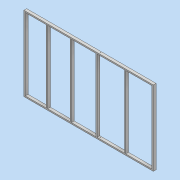
# Autodesk Inventor part: Khung cửa
Saved by Autodesk Inventor 2018 (Build 220112000, 112)
## iProperties
Created: 2020-08-10
Part Number: Khung cửa
Material: Generic
Document SubType Name: Modeling
Designer: ASUS
Density: 1 g/cm^3
Appearance: Default
Author: ASUS
Autodesk Inventor part; units mm, degrees
ref_plane "YZ Plane" through (0, 0, 0) normal (1, 0, 0) x (0, 1, 0)
ref_plane "XZ Plane" through (0, 0, 0) normal (0, 1, 0) x (-1, 0, 0)
ref_plane "XY Plane" through (0, 0, 0) normal (0, 0, 1) x (1, 0, 0)
sketch "Sketch1" plane through (0, 0, 0) normal (0, 1, 0) x (-1, 0, 0)
  line L0 (0, 0) -> (2835, 0)
  line L1 (2835, 0) -> (2835, -1640)
  line L2 (2835, -1640) -> (0, -1640)
  line L3 (0, -1640) -> (0, 0)
  line L4 (30, -30) -> (30, -1610)
  line L5 (2805, -1610) -> (2805, -30)
  line L6 (1232.5, -30) -> (1232.5, -1610)
  line L7 (1262.5, -1610) -> (1262.5, -30)
  line L8 (605, -30) -> (605, -1610)
  line L9 (635, -1610) -> (635, -30)
  line L10 (2315, -30) -> (2315, -1610)
  line L11 (2345, -1610) -> (2345, -30)
  line L12 (1825, -30) -> (1825, -1610)
  line L13 (1795, -1610) -> (1795, -30)
  line L14 (605, -30) -> (30, -30)
  line L15 (30, -1610) -> (605, -1610)
  line L16 (635, -1610) -> (1232.5, -1610)
  line L17 (1232.5, -30) -> (635, -30)
  line L18 (1795, -30) -> (1262.5, -30)
  line L19 (1262.5, -1610) -> (1795, -1610)
  line L20 (2805, -30) -> (2345, -30)
  line L21 (2315, -30) -> (1825, -30)
  line L22 (1825, -1610) -> (2315, -1610)
  line L23 (2345, -1610) -> (2805, -1610)
  dimension "d0" = 2835
  dimension "d1" = 1640
  dimension "d3" = 30
  dimension "d5" = 30
  dimension "d6" = 30
  dimension "d7" = 1262.5
  dimension "d8" = 30
  dimension "d9" = 635
  dimension "d10" = 30
  dimension "d11" = 30
  dimension "d12" = 520
  dimension "d13" = 1040
  constraints: 48 end point, 32 parallel, 6 horizontal, 6 perpendicular
  measures "d0" distance of L1.end L2.end
  measures "d1" distance of L0.end L1.end
  measures "d3" distance between parallel lines of L1 L5
  measures "d5" distance between parallel lines of L3 L4
  measures "d6" distance between parallel lines of L6 L7
  measures "d7" distance between parallel lines of L3 L7
  measures "d8" distance between parallel lines of L8 L9
  measures "d9" distance between parallel lines of L3 L9
  measures "d10" distance of L11.start L10.end
  measures "d11" distance between parallel lines of L13 L12
  measures "d12" distance between parallel lines of L1 L10
  measures "d13" distance between parallel lines of L13 L1
extrude "Extrusion1" add sketch "Sketch1" along normal blind 60
sketch "Sketch2" plane through (-2835, 0, 0) normal (0, 0, 1) x (1, 0, 0)
  circle A0 centre (1642.5, 30) radius 5
  line L0 (2835, 0) -> (0, 0) projected
  point P0 (1602.5, 60)
  dimension "d16" = 10
  dimension "d17" = 30
  dimension "d18" = 40
  constraints: 1 centre point
  measures "d16" diameter of A0
  measures "d17" distance from line of L0 A0.centre
  measures "d18" horizontal distance of point (1602.5, 60) A0.centre
extrude "Extrusion2" cut sketch "Sketch2" against normal blind 3000
body "Solid1"
